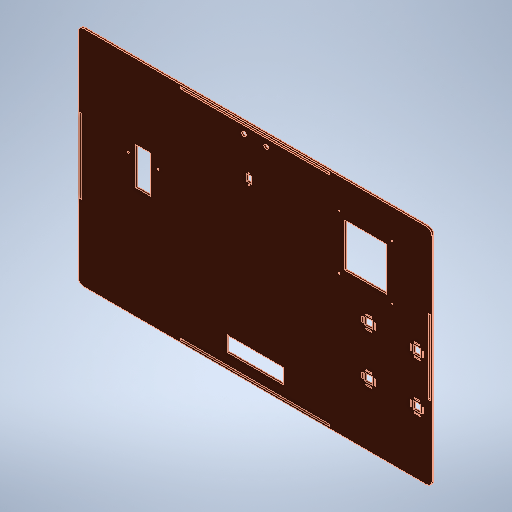
# Autodesk Inventor part: Table
Saved by Autodesk Inventor 2025.4 (Build 294407000, 407)
## iProperties
Created: 2026-04-11
Part Number: Table
Material: Generic
Document SubType Name: Sheet Metal
Designer: lenovo
Density: 1 g/cm^3
Sheet Metal Rule: Default_mm
Appearance: Default(1)
Author: lenovo
Autodesk Inventor part; units mm, degrees
ref_plane "YZ Plane" through (0, 0, 0) normal (1, 0, 0) x (0, 1, 0)
ref_plane "XZ Plane" through (0, 0, 0) normal (0, 1, 0) x (-1, 0, 0)
ref_plane "XY Plane" through (0, 0, 0) normal (0, 0, 1) x (1, 0, 0)
sketch "Sketch1" plane through (0, 0, 0) normal (0, 0, 1) x (1, 0, 0)
  line L0 (-475, -300) -> (475, -300)
  line L1 (475, -300) -> (475, 300)
  line L2 (475, 300) -> (-475, 300)
  line L3 (-475, 300) -> (-475, -300)
  line L4 (-475, -300) -> (475, 300) construction
  line L5 (475, -300) -> (-475, 300) construction
  point P0 (0, 0)
  dimension "d0" = 950
  dimension "d1" = 600
  measures "d0" distance of L2.end L1.end
  measures "d1" distance of L1.end L0.end
extrude "Plate1" add sketch "Sketch1" along normal blind 5
sketch "Sketch4" plane through (0, 0, 5) normal (0, 0, 1) x (1, 0, 0)
  circle A0 centre (-340, 72) radius 2.15
  circle A1 centre (-260, 72) radius 2.15
  line L0 (-475, 300) -> (475, 300) projected
  line L1 (475, 300) -> (475, -300) projected
  line L2 (-280, 0) -> (-320, 0)
  line L3 (-320, 0) -> (-320, 100)
  line L4 (-320, 100) -> (-280, 100)
  line L5 (-280, 100) -> (-280, 0)
  line L6 (-475, -300) -> (-475, 300) projected
  point P0 (0, 0)
  point P1 (-300, 0)
  dimension "d18" = 4.3
  dimension "d19" = 228
  dimension "d21" = 80
  dimension "d22" = 40
  dimension "d23" = 40
  dimension "d24" = 100
  dimension "d27" = 135
  constraints: 8 end point, 2 centre point, 2 horizontal alignment, 2 parallel, 1 equal radius, 1 horizontal, 1 midpoint, 1 perpendicular
  measures "d18" diameter of A1
  measures "d19" distance from line of L0 A1.centre
  measures "d21" distance of A0.centre A1.centre
  measures "d22" horizontal distance of A1.centre point (-300, 0)
  measures "d23" distance between parallel lines of L3 L5
  measures "d24" distance of L2.end L3.end
  measures "d27" distance from line of L6 A0.centre
extrude "Sorting Fixation" cut sketch "Sketch4" against normal blind 5
sketch "Sketch5" plane through (0, 0, 0) normal (0, 0, -1) x (-1, 0, 0)
  line L0 (-265, -172.134) -> (-475, -172.134) construction
  line L1 (-475, -172.134) -> (-475, 37.866) construction
  line L2 (-475, 37.866) -> (-265, 37.866) construction
  line L3 (-265, 37.866) -> (-265, -172.134) construction
  line L4 (-475, -300) -> (-475, 300) projected
  line L5 (475, -300) -> (-475, -300) projected
  line L6 (-475, -172.134) -> (-435, -172.134)
  line L7 (-435, -172.134) -> (-435, -132.134)
  line L8 (-435, -132.134) -> (-475, -132.134)
  line L9 (-475, -132.134) -> (-475, -172.134)
  line L10 (-425, -122.134) -> (-445, -122.134)
  line L11 (-445, -122.134) -> (-445, -142.134)
  line L12 (-445, -142.134) -> (-425, -142.134)
  line L13 (-425, -142.134) -> (-425, -122.134)
  line L14 (-425, -122.134) -> (-445, -142.134) construction
  line L15 (-445, -122.134) -> (-425, -142.134) construction
  line L16 (-450, -124.634) -> (-453.08, -124.634)
  line L17 (-453.08, -124.634) -> (-453.08, -139.634)
  line L18 (-453.08, -139.634) -> (-450, -139.634)
  line L19 (-450, -139.634) -> (-450, -124.634)
  line L20 (-450, -124.634) -> (-453.08, -139.634) construction
  line L21 (-453.08, -124.634) -> (-450, -139.634) construction
  line L22 (-420, -124.634) -> (-416.92, -124.634)
  line L23 (-416.92, -124.634) -> (-416.92, -139.634)
  line L24 (-416.92, -139.634) -> (-420, -139.634)
  line L25 (-420, -139.634) -> (-420, -124.634)
  line L26 (-420, -124.634) -> (-416.92, -139.634) construction
  line L27 (-416.92, -124.634) -> (-420, -139.634) construction
  line L28 (-427.5, -150.214) -> (-442.5, -150.214)
  line L29 (-442.5, -150.214) -> (-442.5, -147.134)
  line L30 (-442.5, -147.134) -> (-427.5, -147.134)
  line L31 (-427.5, -147.134) -> (-427.5, -150.214)
  line L32 (-427.5, -150.214) -> (-442.5, -147.134) construction
  line L33 (-442.5, -150.214) -> (-427.5, -147.134) construction
  line L34 (-427.5, -114.054) -> (-442.5, -114.054)
  line L35 (-442.5, -114.054) -> (-442.5, -117.134)
  line L36 (-442.5, -117.134) -> (-427.5, -117.134)
  line L37 (-427.5, -117.134) -> (-427.5, -114.054)
  line L38 (-265, -67.134) -> (-475, -67.134)
  line L39 (-370, -172.134) -> (-370, 37.866)
  line L40 (-265, -172.134) -> (-265, 37.866) construction
  line L41 (-315, -122.134) -> (-295, -122.134)
  line L42 (-295, -122.134) -> (-295, -142.134)
  line L43 (-295, -142.134) -> (-315, -142.134)
  line L44 (-315, -142.134) -> (-315, -122.134)
  line L45 (-315, -122.134) -> (-295, -142.134) construction
  line L46 (-295, -122.134) -> (-315, -142.134) construction
  line L47 (-290, -124.634) -> (-286.92, -124.634)
  line L48 (-286.92, -124.634) -> (-286.92, -139.634)
  line L49 (-286.92, -139.634) -> (-290, -139.634)
  line L50 (-290, -139.634) -> (-290, -124.634)
  line L51 (-290, -124.634) -> (-286.92, -139.634) construction
  line L52 (-286.92, -124.634) -> (-290, -139.634) construction
  line L53 (-320, -124.634) -> (-323.08, -124.634)
  line L54 (-323.08, -139.634) -> (-320, -139.634)
  line L55 (-320, -124.634) -> (-323.08, -139.634) construction
  line L56 (-323.08, -124.634) -> (-320, -139.634) construction
  line L57 (-323.08, -124.634) -> (-323.08, -139.634)
  line L58 (-320, -139.634) -> (-320, -124.634)
  line L59 (-312.5, -150.214) -> (-297.5, -150.214)
  line L60 (-297.5, -150.214) -> (-297.5, -147.134)
  line L61 (-297.5, -147.134) -> (-312.5, -147.134)
  line L62 (-312.5, -147.134) -> (-312.5, -150.214)
  line L63 (-312.5, -150.214) -> (-297.5, -147.134) construction
  line L64 (-297.5, -150.214) -> (-312.5, -147.134) construction
  line L65 (-297.5, -114.054) -> (-297.5, -117.134)
  line L66 (-312.5, -117.134) -> (-312.5, -114.054)
  line L67 (-297.5, -117.134) -> (-312.5, -117.134)
  line L68 (-312.5, -114.054) -> (-297.5, -114.054)
  line L69 (-425, -12.134) -> (-445, -12.134)
  line L70 (-445, -12.134) -> (-445, 7.866)
  line L71 (-445, 7.866) -> (-425, 7.866)
  line L72 (-425, 7.866) -> (-425, -12.134)
  line L73 (-425, -12.134) -> (-445, 7.866) construction
  line L74 (-445, -12.134) -> (-425, 7.866) construction
  line L75 (-450, -9.634) -> (-453.08, -9.634)
  line L76 (-453.08, -9.634) -> (-453.08, 5.366)
  line L77 (-453.08, 5.366) -> (-450, 5.366)
  line L78 (-450, 5.366) -> (-450, -9.634)
  line L79 (-450, -9.634) -> (-453.08, 5.366) construction
  line L80 (-453.08, -9.634) -> (-450, 5.366) construction
  line L81 (-420, -9.634) -> (-416.92, -9.634)
  line L82 (-416.92, 5.366) -> (-420, 5.366)
  line L83 (-420, -9.634) -> (-416.92, 5.366) construction
  line L84 (-416.92, -9.634) -> (-420, 5.366) construction
  line L85 (-416.92, -9.634) -> (-416.92, 5.366)
  line L86 (-420, 5.366) -> (-420, -9.634)
  line L87 (-427.5, 15.946) -> (-442.5, 15.946)
  line L88 (-442.5, 15.946) -> (-442.5, 12.866)
  line L89 (-442.5, 12.866) -> (-427.5, 12.866)
  line L90 (-427.5, 12.866) -> (-427.5, 15.946)
  line L91 (-427.5, 15.946) -> (-442.5, 12.866) construction
  line L92 (-442.5, 15.946) -> (-427.5, 12.866) construction
  line L93 (-442.5, -20.214) -> (-442.5, -17.134)
  line L94 (-427.5, -17.134) -> (-427.5, -20.214)
  line L95 (-442.5, -17.134) -> (-427.5, -17.134)
  line L96 (-427.5, -20.214) -> (-442.5, -20.214)
  line L97 (-315, -12.134) -> (-295, -12.134)
  line L98 (-295, -12.134) -> (-295, 7.866)
  line L99 (-295, 7.866) -> (-315, 7.866)
  line L100 (-315, -12.134) -> (-295, 7.866) construction
  line L101 (-295, -12.134) -> (-315, 7.866) construction
  line L102 (-297.5, 12.866) -> (-312.5, 12.866)
  line L103 (-312.5, 12.866) -> (-312.5, 15.946)
  line L104 (-312.5, 15.946) -> (-297.5, 12.866) construction
  line L105 (-297.5, 15.946) -> (-312.5, 12.866) construction
  line L106 (-297.5, 15.946) -> (-297.5, 12.866)
  line L107 (-312.5, 15.946) -> (-297.5, 15.946)
  line L108 (-323.08, 5.366) -> (-320, 5.366)
  line L109 (-297.5, -17.134) -> (-312.5, -17.134)
  line L110 (-312.5, -20.214) -> (-297.5, -20.214)
  line L111 (-297.5, -20.214) -> (-297.5, -17.134)
  line L112 (-312.5, -17.134) -> (-312.5, -20.214)
  line L113 (-320, 5.366) -> (-320, -9.634)
  line L114 (-323.08, -9.634) -> (-323.08, 5.366)
  line L115 (-320, -9.634) -> (-323.08, -9.634)
  line L116 (-323.08, -9.634) -> (-320, 5.366) construction
  line L117 (-320, -9.634) -> (-323.08, 5.366) construction
  line L118 (-315, 7.866) -> (-315, -12.134)
  line L119 (-290, 5.366) -> (-290, -9.634)
  line L120 (-290, -9.634) -> (-286.92, -9.634)
  line L121 (-286.92, -9.634) -> (-286.92, 5.366)
  line L122 (-286.92, 5.366) -> (-290, 5.366)
  line L123 (-290, -9.634) -> (-286.92, 5.366) construction
  line L124 (-286.92, -9.634) -> (-290, 5.366) construction
  point P0 (0, 0)
  point P1 (-475, 0)
  point P2 (-451.54, -132.134)
  point P3 (-418.46, -132.134)
  point P4 (-435, -148.674)
  point P5 (-435, -115.594)
  point P6 (-435, -117.134)
  point P7 (-435, -147.134)
  point P8 (-305, -132.134)
  point P9 (-288.46, -132.134)
  point P10 (-321.54, -132.134)
  point P11 (-305, -148.674)
  point P12 (-305, -115.594)
  point P13 (-305, -117.134)
  point P14 (-305, -147.134)
  point P15 (-435, -2.134)
  point P16 (-451.54, -2.134)
  point P17 (-418.46, -2.134)
  point P18 (-435, 14.406)
  point P19 (-435, -18.674)
  point P20 (-435, -17.134)
  point P21 (-435, 12.866)
  point P22 (-305, 12.866)
  point P23 (-305, 14.406)
  point P24 (-305, -2.134)
  point P25 (-321.54, -2.134)
  point P26 (-305, -17.134)
  point P27 (-305, -18.674)
  point P28 (-288.46, -2.134)
  dimension "d28" = 210
  dimension "d29" = 127.866
  dimension "d30" = 40
  dimension "d32" = 20
  dimension "d35" = 3.08
  dimension "d36" = 15
  dimension "d37" = 30
  dimension "d38" = 15
  dimension "d39" = 3.08
  dimension "d40" = 30
  constraints: 246 end point, 91 symmetric about line, 13 midpoint, 10 parallel, 9 perpendicular, 5 horizontal, 2 point on line, 1 vertical alignment
  measures "d28" distance of L0.start L0.end
  measures "d29" distance between parallel lines of L5 L0
  measures "d30" distance of L8.end L7.end
  measures "d32" distance of L12.end L11.end
  measures "d35" distance of L18.end L17.end
  measures "d36" distance of L17.end L16.end
  measures "d37" distance between parallel lines of L25 L19
  measures "d38" distance of L29.end L30.end
  measures "d39" distance of L28.end L29.end
  measures "d40" distance of point (-435, -117.134) point (-435, -147.134)
extrude "Shooting Fixation" cut sketch "Sketch5" against normal blind 5 contours L17 L16 L19 L8 | L8 L19 L18 L17 | L28 L29 L30 L7 | L7 L30 L31 L28 | L11 L10 L13 L12 L7 L8 | L8 L7 L12 L11 | L22 L23 L24 L25 | L37 L36 L35 L34 | L41 L42 L43 L44 | L47 L48 L49 L50 | L58 L54 L57 L53 | L62 L61 L60 L59 | L65 L67 L66 L68 | L69 L70 L71 L72 | L75 L76 L77 L78 | L86 L82 L85 L81 | L90 L89 L88 L87 | L93 L95 L94 L96 | L118 L99 L98 L97 | L102 L103 L107 L106 | L108 L113 L115 L114 | L111 L110 L112 L109 | L122 L121 L120 L119
sketch "Sketch6" plane through (0, 0, 5) normal (0, 0, 1) x (1, 0, 0)
  line L0 (-475, 300) -> (-475, -300) projected
  line L1 (-475, 0) -> (475, 0)
  line L2 (475, -300) -> (475, 300) projected
  line L3 (475, 300) -> (-475, 300) projected
  line L4 (0, 300) -> (0, -300)
  line L5 (475, -300) -> (-475, -300) projected
  line L6 (-200, 295) -> (200, 295)
  line L7 (200, 295) -> (200, 289.92)
  line L8 (200, 289.92) -> (-200, 289.92)
  line L9 (-200, 289.92) -> (-200, 295)
  line L10 (-200, 295) -> (200, 289.92) construction
  line L11 (200, 295) -> (-200, 289.92) construction
  line L12 (-475, 300) -> (475, 300) projected
  line L13 (-470, -100) -> (-464.92, -100)
  line L14 (-464.92, -100) -> (-464.92, 100)
  line L15 (-464.92, 100) -> (-470, 100)
  line L16 (-470, 100) -> (-470, -100)
  line L17 (-470, -100) -> (-464.92, 100) construction
  line L18 (-464.92, -100) -> (-470, 100) construction
  line L19 (-475, -300) -> (-475, 300) projected
  line L20 (-200, -295) -> (200, -295)
  line L21 (200, -295) -> (200, -289.92)
  line L22 (200, -289.92) -> (-200, -289.92)
  line L23 (-200, -289.92) -> (-200, -295)
  line L24 (-200, -295) -> (200, -289.92) construction
  line L25 (200, -295) -> (-200, -289.92) construction
  line L26 (470, -100) -> (464.92, -100)
  line L27 (464.92, -100) -> (464.92, 100)
  line L28 (464.92, 100) -> (470, 100)
  line L29 (470, 100) -> (470, -100)
  line L30 (470, -100) -> (464.92, 100) construction
  line L31 (464.92, -100) -> (470, 100) construction
  point P0 (0, 0)
  point P1 (0, 292.46)
  point P2 (0, 295)
  point P3 (-467.46, 0)
  point P4 (-470, 0)
  point P5 (0, -300)
  point P6 (0, -292.46)
  point P7 (0, -300)
  point P8 (0, -295)
  point P9 (475, 0)
  point P10 (467.46, 0)
  point P11 (475, 0)
  point P12 (470, 0)
  dimension "d43" = 5.08
  dimension "d44" = 400
  dimension "d46" = 5
  dimension "d47" = 5.08
  dimension "d48" = 200
  dimension "d49" = 5
  constraints: 52 end point, 16 symmetric about line, 12 midpoint, 4 parallel, 2 horizontal, 2 perpendicular, 2 point on line, 1 vertical
  measures "d43" distance between parallel lines of L6 L8
  measures "d44" distance of L6.start L6.end
  measures "d46" distance of point (0, 300) point (0, 295)
  measures "d47" distance of L15.end L14.end
  measures "d48" distance of L14.end L13.end
  measures "d49" distance of point (-475, 0) point (-470, 0)
extrude "Side Wall Slots" cut sketch "Sketch6" against normal blind 5 contours L16 L15 L14 L1 | L1 L14 L13 L16 | L6 L7 L8 L4 | L4 L8 L9 L6 | L20 L23 L22 L4 | L4 L22 L21 L20 | L29 L26 L27 L1 | L1 L27 L28 L29
fillet "Corner Round1" radius 15 4 edges at (-475, 300, 2.5) (475, 300, 2.5) (475, -300, 2.5) (-475, -300, 2.5)
sketch "Sketch7" plane through (0, 0, 0) normal (0, 0, -1) x (-1, 0, 0)
  line L0 (-226, 74) -> (-368, 74)
  line L1 (-368, 74) -> (-368, 220)
  line L2 (-368, 220) -> (-226, 220)
  line L3 (-226, 220) -> (-226, 74)
  line L4 (-475, -285) -> (-475, 285) projected
  line L5 (-460, 300) -> (460, 300) projected
  circle A0 centre (-368, 74) radius 1.6
  circle A1 centre (-368, 220) radius 1.6
  circle A2 centre (-226, 220) radius 1.6
  circle A3 centre (-226, 74) radius 1.6
  line L6 (-241, 89) -> (-353, 89)
  line L7 (-353, 89) -> (-353, 205)
  line L8 (-353, 205) -> (-241, 205)
  line L9 (-241, 205) -> (-241, 89)
  point P0 (0, 0)
  dimension "d53" = 142
  dimension "d54" = 146
  dimension "d55" = 107
  dimension "d56" = 80
  dimension "d57" = 3.2
  dimension "d58" = 3.2
  dimension "d59" = 3.2
  dimension "d60" = 3.2
  dimension "d63" = 15
  constraints: 16 end point, 4 centre point, 4 coincident, 4 parallel, 2 perpendicular, 1 horizontal, 3 other
  measures "d53" distance of L1.end L2.end
  measures "d54" distance of L0.end L1.end
  measures "d55" distance between parallel lines of L4 L1
  measures "d56" distance between parallel lines of L5 L2
  measures "d57" diameter of A0
  measures "d58" diameter of A1
  measures "d59" diameter of A2
  measures "d60" diameter of A3
  measures "d63" distance between parallel lines of L3 L9
extrude "Lifting Fixation" cut sketch "Sketch7" against normal blind 5 contours A0 L1 L0 | L0 L1 A0 | A3 L3 L0 | L0 L3 A3 | A1 L2 L1 | L1 L2 A1 | A2 L2 L3 | L3 L2 A2 | L6 L7 L8 L9
sketch "Sketch8" plane through (0, 0, 0) normal (0, 0, -1) x (-1, 0, 0)
  circle A0 centre (16.374, 185.35) radius 1.6
  line L0 (-460, 300) -> (460, 300) projected
  line L1 (475, 285) -> (475, -285) projected
  circle A1 centre (16.374, 158.35) radius 1.6
  line L2 (8.874, 181.35) -> (23.874, 181.35)
  line L3 (23.874, 181.35) -> (23.874, 163.35)
  line L4 (23.874, 163.35) -> (8.874, 163.35)
  line L5 (8.874, 163.35) -> (8.874, 181.35)
  line L6 (8.874, 181.35) -> (23.874, 163.35) construction
  line L7 (23.874, 181.35) -> (8.874, 163.35) construction
  point P0 (0, 0)
  point P1 (16.374, 172.35)
  dimension "d64" = 3.2
  dimension "d65" = 114.65
  dimension "d66" = 458.626
  dimension "d67" = 3.2
  dimension "d68" = 27
  dimension "d82" = 18
  dimension "d83" = 15
  dimension "d84" = 4
  constraints: 12 end point, 2 centre point, 2 midpoint, 2 parallel, 2 vertical alignment, 1 horizontal, 1 perpendicular
  measures "d64" diameter of A0
  measures "d65" distance from line of L0 A0.centre
  measures "d66" distance from line of L1 A0.centre
  measures "d67" diameter of A1
  measures "d68" distance of A0.centre A1.centre
  measures "d82" distance of L2.end L3.end
  measures "d83" distance of L3.end L4.end
  measures "d84" distance from line of A0.centre L2
extrude "Cut7" cut sketch "Sketch8" against normal blind 5
sketch "Sketch9" plane through (0, 0, 0) normal (0, 0, -1) x (-1, 0, 0)
  line L0 (-75, -260) -> (75, -260)
  line L1 (75, -260) -> (75, -220)
  line L2 (75, -220) -> (-75, -220)
  line L3 (-75, -220) -> (-75, -260)
  line L4 (-75, -260) -> (75, -220) construction
  line L5 (75, -260) -> (-75, -220) construction
  point P0 (0, 0)
  point P1 (0, -240)
  dimension "d71" = 150
  dimension "d72" = 40
  dimension "d73" = 240
  constraints: 12 end point, 2 midpoint, 2 parallel, 1 horizontal, 1 perpendicular, 1 vertical alignment
  measures "d71" distance of L2.end L1.end
  measures "d72" distance of L1.end L0.end
  measures "d73" distance of point (0, -240) point (0, 0)
extrude "Cut8" cut sketch "Sketch9" against normal blind 5
sketch "Sketch10" plane through (0, 0, 0) normal (0, 0, -1) x (-1, 0, 0)
  line L0 (0, 0) -> (0, 300)
  line L1 (-460, 300) -> (460, 300) projected
  circle A0 centre (30, 269.92) radius 6.125
  line L2 (200, 289.92) -> (-200, 289.92) projected
  circle A1 centre (-30, 269.92) radius 6.125
  dimension "d76" = 12.25
  dimension "d77" = 20
  dimension "d78" = 60
  constraints: 2 centre point, 2 end point, 1 midpoint, 1 symmetric about line, 1 vertical, 1 other
  measures "d76" diameter of A0
  measures "d77" distance from line of A0.centre L2
  measures "d78" diameter of A0.centre L0
extrude "Cut9" cut sketch "Sketch10" against normal blind 5
equation "\"d25\" = Thickness"
equation "\"d40\" = d37"
equation "\"d41\" = Thickness"
equation "\"d50\" = Thickness"
equation "\"d61\" = Thickness"
equation "\"d69\" = Thickness"
equation "\"d74\" = Thickness"
equation "\"d79\" = Thickness"
equation "\"d2\" = Thickness"
equation "\"BendRadius\" = Thickness"
equation "\"BendReliefWidth\" = Thickness"
equation "\"BendReliefDepth\" = 0.5 * Thickness"
equation "\"TransitionRadius\" = BendRadius"
equation "\"JacobiRadiusSize\" = BendRadius"
equation "\"GapSize\" = Thickness"
equation "\"Thickness\" = 5"
body "Solid1"
